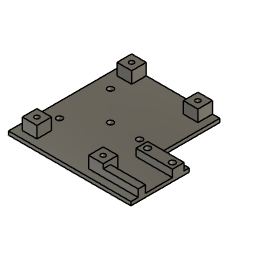
mount_board (Autodesk Fusion 360 design; units mm, degrees)
Autodesk Fusion 360 part; units mm, degrees
box "BoxPrimitive1" add length 80 width 80 height 2.5 placed x (0, 1, 0) y (-1, 0, 0) z (0, 0, 1) at (85, 5, 0)
box "BoxPrimitive2" add length 10 width 10 height 5 placed x (0, 1, 0) y (-1, 0, 0) z (0, 0, 1) at (20, 10, 2.5)
box "BoxPrimitive3" add length 10 width 10 height 5 placed x (0, 1, 0) y (-1, 0, 0) z (0, 0, 1) at (20, 70, 2.5)
extrude "Extrude1" add 1 faces at (16.6667, 80, 4.1667) along direction (0, 1, 0) blind 5
extrude "Extrude2" cut 1 faces at (16.6667, 70, 4.1667) along direction (0, 1, 0) blind 5
box "BoxPrimitive4" add length 10 width 10 height 5 placed x (0, 1, 0) y (-1, 0, 0) z (0, 0, 1) at (65, 10, 0)
extrude "Extrude3" add 1 faces at (58.3333, 13.3333, 5) along direction (0, 0, 1) blind 5
extrude "Extrude4" cut 1 faces at (58.3333, 13.3333, 10) along direction (0, 0, -1) blind 2.5
box "BoxPrimitive5" add length 10 width 10 height 7.5 placed x (0, 1, 0) y (-1, 0, 0) z (0, 0, 1) at (65, 75, 0)
extrude "Extrude5" cut 1 faces at (85, 58.3333, 0.8333) along direction (-1, 0, 0) blind 15
extrude "Extrude6" add 1 faces at (70, 58.3333, 0.8333) along direction (1, 0, 0) blind 15
box "BoxPrimitive6" add length 5 width 20 height 5 placed x (0, -1, 0) y (1, 0, 0) z (0, 0, 1) at (65, 40, 2.5)
box "BoxPrimitive7" add length 5 width 20 height 5 placed x (0, 1, 0) y (-1, 0, 0) z (0, 0, 1) at (85, 10, 0)
extrude "Extrude7" add 1 faces at (58.3333, 13.3333, 7.5) along direction (0, 0, 1) blind 3
extrude "Extrude8" add 1 faces at (13.3333, 13.3333, 7.5) along direction (0, 0, 1) blind 3
extrude "Extrude9" add 1 faces at (58.3333, 78.3333, 7.5) along direction (0, 0, 1) blind 3
extrude "Extrude10" add 1 faces at (13.3333, 81.6667, 7.5) along direction (0, 0, 1) blind 3
extrude "Extrude11" add 1 faces at (71.6667, 11.6667, 5) along direction (0, 0, 1) blind 2.5
extrude "Extrude12" add 1 faces at (85, 11.6667, 4.1667) along direction (1, 0, 0) blind 10
hole "Hole5" at (68, 37.5, 7.5) direction (0, 0, -1) diameter 4 depth 5 tip angle 180
extrude "Extrude13" cut 1 faces at (95, 11.6667, 4.1667) along direction (-1, 0, 0) blind 7
extrude "Extrude14" add 1 faces at (72.6667, 35, 4.1667) along direction (0, -1, 0) blind 1
extrude "Extrude15" add 1 faces at (72.6667, 40, 4.1667) along direction (0, 1, 0) blind 1
extrude "Extrude16" cut 1 faces at (88, 36.3333, 4.1667) along direction (-1, 0, 0) blind 1
hole "Hole7" at (60, 80, 10.5) direction (0, 0, -1) diameter 3.2 depth 5 tip angle 180
hole "Hole8" at (15, 80, 10.5) direction (0, 0, -1) diameter 3.2 depth 5 tip angle 180
hole "Hole9" at (60, 15, 10.5) direction (0, 0, -1) diameter 3.2 depth 5 tip angle 180
hole "Hole10" at (15, 15, 10.5) direction (0, 0, -1) diameter 3.2 depth 5 tip angle 180
hole "Hole11" at (35, 45, 2.5) direction (0, 0, -1) diameter 4 depth 5 tip angle 180
hole "Hole12" at (55, 45, 2.5) direction (0, 0, -1) diameter 4 depth 5 tip angle 180
extrude "Extrude17" add 1 faces at (65, 36.3333, 4.1667) along direction (-1, 0, 0) blind 1
extrude "Extrude18" add 1 faces at (87, 36.3333, 4.1667) along direction (1, 0, 0) blind 1
extrude "Extrude19" add 1 faces at (80, 41, 5.8333) along direction (0, 1, 0) blind 0.5
extrude "Extrude20" add 1 faces at (72, 34, 4.1667) along direction (0, -1, 0) blind 0.5
hole "Hole13" at (15, 65, 2.5) direction (0, 0, -1) diameter 4 depth 12 tip angle 180
hole "Hole14" at (15, 30, 2.5) direction (0, 0, -1) diameter 4 depth 12 tip angle 180
extrude "Extrude21" add 1 faces at (88, 36.1667, 5.8333) along direction (1, 0, 0) blind 1
hole "Hole15" at (85, 37.5, 7.5) direction (0, 0, -1) diameter 4 depth 5 tip angle 180
sketch "Sketch10" plane through (0, 0, 2.5) normal (0, 0, 1) x (-1, 0, 0)
  circle A0 centre (-15, -30) radius 2
  circle A1 centre (-15, -65) radius 2
  line L0 (-64, -33.5) -> (-64, -41.5)
  line L1 (-64, -41.5) -> (-89, -41.5)
  line L2 (-89, -41.5) -> (-89, -85)
  line L3 (-89, -85) -> (-65, -85)
  line L4 (-65, -85) -> (-65, -75)
  line L5 (-65, -75) -> (-55, -75)
  line L6 (-55, -75) -> (-55, -85)
  line L7 (-55, -85) -> (-20, -85)
  line L8 (-20, -85) -> (-20, -75)
  line L9 (-20, -75) -> (-10, -75)
  line L10 (-10, -75) -> (-10, -85)
  line L11 (-10, -85) -> (-5, -85)
  line L12 (-5, -85) -> (-5, -5)
  line L13 (-5, -5) -> (-89, -5)
  line L14 (-89, -5) -> (-89, -10)
  line L15 (-89, -10) -> (-55, -10)
  line L16 (-55, -10) -> (-55, -20)
  line L17 (-55, -20) -> (-65, -20)
  line L18 (-65, -20) -> (-65, -15)
  line L19 (-65, -15) -> (-89, -15)
  line L20 (-89, -15) -> (-89, -33.5)
  line L21 (-89, -33.5) -> (-64, -33.5)
  circle A2 centre (-55, -45) radius 2
  circle A3 centre (-35, -45) radius 2
  line L22 (-20, -20) -> (-20, -10)
  line L23 (-20, -10) -> (-10, -10)
  line L24 (-10, -10) -> (-10, -20)
  line L25 (-10, -20) -> (-20, -20)
  line L26 (-70, -85) -> (-70, -45)
  line L27 (-70, -45) -> (-89, -45)
  constraint coincident L3 L26.start
  constraint perpendicular L3 L26
  constraint coincident L2 L27.end
  constraint perpendicular L2 L27
extrude "Extrude22" cut sketch "Sketch10" against normal blind 3 contours L2 L3 L26 L27
move_face "MoveFace2" to x (1, 0, 0) y (0, 1, 0) z (0, 0, 1) at (-0.5, 0, 0) 7 faces at (16.6667, 10, 5.1667) (20, 13.3333, 5.1667) (11.1348, 15.0399, 10.5) (15.0798, 13.402, 8.8333) (15.5318, 14.1782, 5.5) (16.6667, 20, 5.1667) (10, 13.3333, 5.1667)
move_face "MoveFace3" to x (1, 0, 0) y (0, 1, 0) z (0, 0, 1) at (-0.5, 0, 0) 7 faces at (10, 78.3333, 7.8333) (61.6667, 85, 7.8333) (18.8652, 79.9601, 10.5) (16.6667, 75, 5.1667) (20, 81.6667, 5.1667) (13.4005, 80.0399, 8.8333) (14.8082, 80.5815, 5.5)
